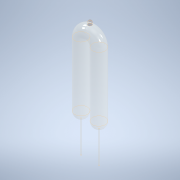
# Autodesk Inventor part: Flashbulb-DU8902
Saved by Autodesk Inventor 2022 (Build 260153000, 153)
## iProperties
Created: 2021-10-25
Part Number: Flashbulb-DU8902
Material: Phenolic Resin
Document SubType Name: Modeling
Designer: incep
Density: 1.38 g/cm^3
Appearance: Polycarbonate - Smoked
Author: incep
Autodesk Inventor part; units mm, degrees
ref_plane "YZ Plane" through (0, 0, 0) normal (1, 0, 0) x (0, 1, 0)
ref_plane "XY Plane" through (0, 0, 0) normal (0, 0, 1) x (1, 0, 0)
sketch "Sketch1" plane through (0, 0, 0) normal (0, 1, 0) x (-1, 0, 0)
  circle A0 centre (7, 0) radius 5
  circle A1 centre (-7, 0) radius 5
  line L0 (7, 0) -> (-7, 0) construction
  line L1 (12, 0) -> (2, 0)
  line L2 (-2, 0) -> (-12, 0)
  circle A2 centre (-7, 0) radius 0.35
  circle A3 centre (7, 0) radius 0.35
  point P0 (0, 0)
  point P1 (0, 0)
  dimension "d0" = 10
  dimension "d1" = 14
  dimension "d8" = 0.7
  constraints: 6 end point, 4 centre point, 4 point on circle, 3 coincident, 3 point on line, 2 equal radius, 1 horizontal, 1 midpoint
  measures "d0" diameter of A0
  measures "d1" distance of L0.end L0.start
  measures "d8" diameter of A3
sketch "Sketch2" plane through (0, 0, 0) normal (0, 0, 1) x (1, 0, 0)
  line L0 (7, 0) -> (7, 50)
  line L1 (-7, 0) -> (-7, 50)
  line L2 (-7, 0) -> (7, 0) construction
  arc A0 (7, 50) -> (-7, 50) centre (0, 50) ccw
  point P0 (0, 0)
  point P1 (0, 0)
  dimension "d2" = 14
  dimension "d3" = 50
  constraints: 6 end point, 2 point on circle, 2 tangent, 2 vertical, 1 centre point, 1 coincident, 1 horizontal, 1 midpoint, 1 parallel
  measures "d2" distance between parallel lines of L0 L1
  measures "d3" distance of point (0, 0) A0.centre
sweep "Sweep1" add profiles "Sketch1" path "Sketch2" contours L2 A2 A1 | A1 L2 A2 | A2 L2 | L2 A2
revolve "Revolution1" add sketch "Sketch1" angle 360 about axis through (-7, 0, 0) along (1, 0, 0) picked at (3.6018, 0.4268) picked at (7.0663, 0.096) contours L1 A3 A0 | L1 A3
revolve "Revolution2" add sketch "Sketch1" angle 360 about axis through (2, 0, 0) along (1, 0, 0) picked at (-10.3982, 0.4268) picked at (-6.9337, 0.096) contours L2 A2 A1 | L2 A2
extrude "Extrusion1" add sketch "Sketch1" against normal blind 30 contours A3 L1 | L1 A3 | A2 L2 | L2 A2
ref_plane "Work Plane1" through (0, 61, 0) normal (0, 1, 0) x (-1, 0, 0)
sketch "Sketch3" plane through (0, 61, 0) normal (0, 1, 0) x (-1, 0, 0)
  circle A0 centre (0, 0) radius 1.5
  dimension "d12" = 3
  constraints: 1 centre point, 1 coincident
  measures "d12" diameter of A0
extrude "Extrusion2" add sketch "Sketch3" along normal blind 4
fillet "Fillet1" radius 1.5 1 edges at (1.5, 65, 0)
body "Solid1"
